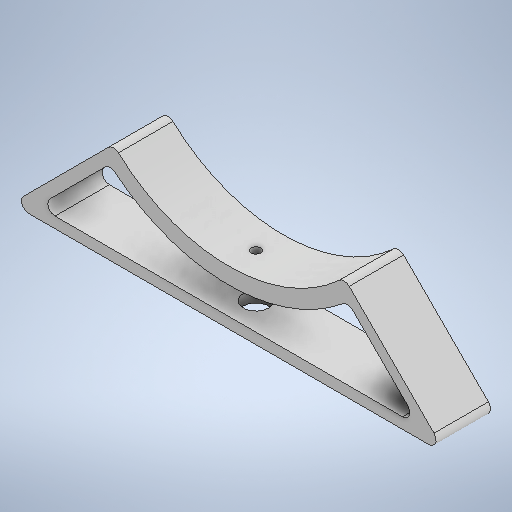
# Autodesk Inventor part: Horizontal Base
Saved by Autodesk Inventor 2025.3 (Build 293356000, 356)
## iProperties
Created: 2025-07-02
Part Number: Horizontal Base
Material: Generic
Document SubType Name: Modeling
Designer: vncnt
Density: 1 g/cm^3
Appearance: Default
Author: vncnt
## iProperties of the stored document Horizontal Base_3DPrint.ipt
Created: 2025-07-02
Part Number: Horizontal Base_3DPrint
Material: Generic
Document SubType Name: Modeling
Designer: vncnt
Density: 1 g/cm^3
Appearance: Default
Author: vncnt
Autodesk Inventor part; units mm, degrees
ref_plane "YZ Plane" through (0, 0, 0) normal (1, 0, 0) x (0, 1, 0)
ref_plane "XZ Plane" through (0, 0, 0) normal (0, 1, 0) x (-1, 0, 0)
ref_plane "XY Plane" through (0, 0, 0) normal (0, 0, 1) x (1, 0, 0)
sketch "Sketch1" plane through (0, 0, 0) normal (0, 0, 1) x (1, 0, 0)
  circle A0 centre (0, 0) radius 45
  line L0 (0, 0) -> (0, -60)
  line L1 (0, -60) -> (60, -60)
  line L2 (60, -60) -> (31.8198, -31.8198)
  line L3 (0, -60) -> (-60, -60)
  line L4 (-60, -60) -> (-31.8198, -31.8198)
  line L5 (29.6985, -33.9411) -> (52.7574, -57)
  line L6 (52.7574, -57) -> (0, -57)
  line L7 (-29.6985, -33.9411) -> (-52.7574, -57)
  line L8 (-52.7574, -57) -> (0, -57)
  circle A1 centre (0, 0) radius 49.5
  point P0 (0, -45)
  point P1 (32.8161, -37.0588)
  point P2 (-32.8161, -37.0588)
  dimension "d0" = 90
  dimension "d1" = 60
  dimension "d2" = 60
  dimension "d3" = 45
  dimension "d18" = 3
  dimension "d19" = 3
  dimension "d20" = 4.5
  constraints: 18 end point, 2 symmetric about line, 1 centre point, 1 coincident, 1 perpendicular, 1 vertical, 5 other
  measures "d1" distance of L0.start L0.end
  measures "d2" distance of L0.end L1.end
  measures "d3" angle of L2 L1
  measures "d18" distance between parallel lines of L2 L5
  measures "d19" distance between parallel lines of L4 L7
extrude "Extrusion1" add sketch "Sketch1" along normal blind 15 contours A0 L0 A1 L4 | L2 A1 L0 A0 | A1 L7 L8 L0 L3 L4 | L2 L1 L0 L6 L5 A1
sketch "Sketch6" plane through (-60, -60, 0) normal (0, -1, 0) x (1, 0, 0)
  circle A0 centre (60, 7.5) radius 3.5
  line L0 (0, 15) -> (120, 15) projected
  point P0 (60, 0)
  dimension "d27" = 7
  dimension "d28" = 7.5
  constraints: 1 centre point
  measures "d27" diameter of A0
  measures "d28" distance from line of L0 A0.centre
extrude "Extrusion6" cut sketch "Sketch6" against normal blind 3
sketch "Sketch7" plane through (-60, -60, 0) normal (0, -1, 0) x (1, 0, 0)
  circle A0 centre (60, 7.5) radius 3.5 projected
  circle A1 centre (60, 7.5) radius 1.25
  point P0 (60, 0)
  dimension "d31" = 2.5
  constraints: 1 centre point, 1 coincident
  measures "d31" diameter of A1
extrude "Extrusion7" cut sketch "Sketch7" against normal blind 21.25 contours A1
chamfer "Chamfer1" distance 2 angle 45 1 edges at (-1.25, -49.4842, 7.5043)
fillet "Fillet1" radius 2 8 edges at (-52.7574, -57, 7.5) (-32.8161, -37.0588, 7.5) (32.8161, -37.0588, 7.5) (52.7574, -57, 7.5) (60, -60, 7.5) (-60, -60, 7.5) (-31.8198, -31.8198, 7.5) (31.8198, -31.8198, 7.5)
body "Solid1"
